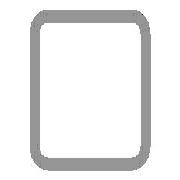
# Autodesk Inventor part: DD_KVD_003_02
Saved by Autodesk Inventor 2017.3 (Build 213256000, 256)
## iProperties
IsCustomPart: 1
Created: 2016-02-22
Part Number: DD_KVD_003_02
Material: Nerezová ocel
Description: Tenkostěnné profily ocelové svařované (čtvercový profil)
Document SubType Name: Plech
Standard: CSN 42 6935
Designer: Darena
Standards Organization: CSN
Language: cs-CZ
Size Designation: 35x35x3-875
Categories: <MemberInstance><Categories><Category DisplayName="Konstrukční profily" InternalName="089c4875-fa83-4c05-b084-43b9cc11f5ed" Mnemonic="GRDR"><CategoryParameter DisplayName="Hmotnost na délkovou jednotku" InternalName="0bb95a10-148f-4027-a459-38d7b056702a" Mnemonic="shpmass"/><CategoryParameter DisplayName="Plocha průřezu" InternalName="1ff91680-64b0-4202-b9a3-7fd3f94bba3b" Mnemonic="secarea"/><CategoryParameter DisplayName="Poloměr setrvačnosti (x)" InternalName="25778675-03e9-40c1-b6a8-4a9ed693320d" Mnemonic="gyrradx"/><CategoryParameter DisplayName="Modul pružnosti v kroucení" InternalName="26c1ec35-5026-4c63-ad0a-751cf684a536" Mnemonic="torrigmod"/><CategoryParameter DisplayName="Vzdálenost těžiště X-X" InternalName="26c9bdb8-9c79-4b4f-a92e-8e197583c9c4" Mnemonic="grcendistX"/><CategoryParameter DisplayName="Původní ID člena" InternalName="340afe4f-75d7-48d3-ab7d-943f3c3da468" Mnemonic="LegacyMemberID"/><CategoryParameter DisplayName="Délka základny" InternalName="42e34263-8f20-4d0e-ad48-bf1385b87c24" Mnemonic="shplen"/><CategoryParameter DisplayName="Moment setrvačnosti (y)" InternalName="4b9f58ea-bced-460e-81ea-3d29ca5a49e3" Mnemonic="inermomy"/><CategoryParameter DisplayName="Moment setrvačnosti (x)" InternalName="4cd780bc-73d7-43ac-917a-579e5cbd684d" Mnemonic="inermomx"/><CategoryParameter DisplayName="Uživatelský referenční bod" InternalName="4f1d1b73-316d-484b-a3df-9cbabb16eb77" Mnemonic="shpBasePoint"/><CategoryParameter DisplayName="Výška tvaru" InternalName="50274e7d-5ac0-4796-92cb-c59e54983c67" Mnemonic="shpheig"/><CategoryParameter DisplayName="Průřezový modul (y)" InternalName="59eaa5e9-d227-48dc-b6c1-6920f96e0f95" Mnemonic="secmody"/><CategoryParameter DisplayName="Označení průřezu" InternalName="5a64d034-428d-49c8-ba32-7619764de20f" Mnemonic="shpdes"/><CategoryParameter DisplayName="Průřezový modul (x)" InternalName="72cfad18-cf51-4ed4-aaa7-c6b224f8419f" Mnemonic="secmodx"/><CategoryParameter DisplayName="Průřezový modul pružnosti" InternalName="7c55a8dc-8844-49f9-a867-cc677b30ec9a" Mnemonic="torsecmod"/><CategoryParameter DisplayName="Šířka tvaru" InternalName="7c717d54-a18f-4666-b4d4-573cce22c62c" Mnemonic="shpwdth"/><CategoryParameter DisplayName="Druhá tloušťka tvaru" InternalName="9251a8e1-85fd-4e47-af99-afdb762317d9" Mnemonic="shpthick2"/><CategoryParameter DisplayName="Publikované popředí" InternalName="9c666724-f362-4ea7-ac62-f6a007de5c69" Mnemonic="shpFGAuto"/><CategoryParameter DisplayName="Vzdálenost těžiště Y-Y" InternalName="bcc4fb17-7af4-436a-8f8c-d0aa3b0248c5" Mnemonic="grcendistY"/><CategoryParameter DisplayName="Poloměr setrvačnosti (y)" InternalName="bfa18ebe-1636-4dbe-8d42-b263e0b73184" Mnemonic="gyrrady"/><CategoryParameter DisplayName="Tloušťka tvaru" InternalName="d109cf76-8eb4-42fc-9800-4409734adc67" Mnemonic="shpthick"/><CategoryParameter DisplayName="Koeficient deformace ve smyku" InternalName="de4c90c6-aaa8-468f-a335-6737b311b5d3" Mnemonic="shdispc"/><Category DisplayName="Trubky čtvercového/obdélníkového průřezu" InternalName="afc8e2d8-05d6-4609-8807-f98a9b7d2ed0" Mnemonic="SQRSHP"><CategoryParameter DisplayName="Plocha průřezu" InternalName="2f7f79dd-983c-4263-802a-5b6a1495fdc5" Mnemonic="secarea"/><CategoryParameter DisplayName="Průřezový modul (x)" InternalName="50d965a6-04bf-46b9-8ace-861858d348e6" Mnemonic="secmodx"/><CategoryParameter DisplayName="Průřezový modul (y)" InternalName="5106aeac-54a2-4159-a9af-8933dd39dba2" Mnemonic="secmody"/><CategoryParameter DisplayName="Tloušťka tvaru" InternalName="52712fc5-f4ee-4eda-b3f2-6fce82c26419" Mnemonic="shpthick"/><CategoryParameter DisplayName="Moment setrvačnosti (y)" InternalName="55ec8510-8276-4c45-8f10-594e0fee7eb3" Mnemonic="inermomy"/><CategoryParameter DisplayName="Poloměr setrvačnosti (x)" InternalName="56c89926-a299-4389-a862-ac94c9691272" Mnemonic="gyrradx"/><CategoryParameter DisplayName="Poloměr" InternalName="5d8d062c-e28e-41c1-98da-8e5fee36da1a" Mnemonic="shprad"/><CategoryParameter DisplayName="Moment setrvačnosti (x)" InternalName="8c4637b6-6b69-4878-9d5d-26a32185d655" Mnemonic="inermomx"/><CategoryParameter DisplayName="Šířka tvaru" InternalName="8c8a1782-5e80-4d77-858b-304b1c0ad1fd" Mnemonic="shpwdth"/><CategoryParameter DisplayName="Poloměr setrvačnosti (y)" InternalName="fa48a7f5-f030-40f9-a60b-de8a845b7104" Mnemonic="gyrrady"/></Category></Category><Category DisplayName="Typdat" InternalName="23b78d0f-2648-40c6-8793-ca6db495c9e8" Mnemonic="DATATYPE"><CategoryParameter DisplayName="Zobrazovanýnázev" InternalName="05415f3d-3907-474b-a020-eb9d644f4cf3" Mnemonic="DISPLAYNAME"/><CategoryParameter DisplayName="Norma" InternalName="0c0a119c-1e12-4c84-803f-101930972f5e" Mnemonic="STANDARD"/><CategoryParameter DisplayName="Popis" InternalName="13903e3d-64b1-4950-80da-f627842ea37f" Mnemonic="DESCRIPTION"/><CategoryParameter DisplayName="Označení" InternalName="2675968c-4ce5-49e0-a4f5-552d29089031" Mnemonic="DESIGNATION"/><CategoryParameter DisplayName="Výchozí řada" InternalName="2af9ec52-faaa-4026-b378-f9fa4afca842" Mnemonic="DEFAULTROW"/><CategoryParameter DisplayName="Název složky" InternalName="3f06958e-8713-4116-9be7-ed6184ecc97b" Mnemonic="FOLDERNAME"/><CategoryParameter DisplayName="GUID verze" InternalName="45a75005-10b1-4dfc-8d6d-dfe629f0b93c" Mnemonic="REVISIONGUID"/><CategoryParameter DisplayName="Názevsouboru" InternalName="8b46a4cc-9585-4fed-90c3-899f57e09a73" Mnemonic="FILENAME"/><CategoryParameter DisplayName="Normalizační institut" InternalName="8f5914e1-4693-403f-8ab5-d37768198c9d" Mnemonic="STDSORG"/><CategoryParameter DisplayName="Verze rodiny" InternalName="914462f6-6e19-4b14-ba84-155b9680b1d0" Mnemonic="FAMILYREVISION"/><CategoryParameter DisplayName="Revize normy" InternalName="91d5a463-65c2-4fde-b823-3b7fea5e8e17" Mnemonic="STANDARDREVISION"/><CategoryParameter DisplayName="Revize členu" InternalName="a65d44b9-392f-4f4f-857b-e4b3d54996fe" Mnemonic="MEMBERREVISION"/><CategoryParameter DisplayName="Formátoříznutí" InternalName="bc51e27b-3422-4e78-93ef-cec197ddf230" Mnemonic="CLIPFORMAT"/><CategoryParameter DisplayName="Výrobce" InternalName="cd6c7a72-a28a-4e50-99a9-2c7f4e13e5ad" Mnemonic="MANUFACTURER"/><CategoryParameter DisplayName="Internínázev" InternalName="cf1d0246-76d9-4b4a-8305-fa0409afb5c1" Mnemonic="INTERNALNAME"/><CategoryParameter DisplayName="Jemetrický" InternalName="e2385c5b-1ea4-4823-96a8-8de651266ec3" Mnemonic="ISMETRIC"/><Category DisplayName="Díl" InternalName="c0e0b642-3bcb-4cc8-9e80-f96d35c4afa4" Mnemonic="PART"><CategoryParameter DisplayName="Číslo dílu" InternalName="016b6077-bfbe-49bd-92c9-d8d59c39c941" Mnemonic="PARTNUMBER"/><CategoryParameter DisplayName="Skladové číslo" InternalName="4dba7c1c-e26c-444e-836c-b08b433409a8" Mnemonic="STOCKNUMBER"/><CategoryParameter DisplayName="Materiál pera" InternalName="5c9a8adb-dd2b-4535-b97f-0a94a95fe41f" Mnemonic="MATERIALKEY"/><CategoryParameter DisplayName="Materiál" InternalName="818a152a-d3c3-49ca-80ee-df7d91421b8e" Mnemonic="MATERIAL"/></Category></Category><Category DisplayName="Původní mapování DA" InternalName="924fff40-ddd0-4eff-ad42-30e3774ef79e" Mnemonic="LEGACYMAPDA"><CategoryParameter DisplayName="DACookie" InternalName="316934ee-8fe1-4c7a-9c36-f2d79e1add1a" Mnemonic="DACOOKIE"/></Category></Categories><FamilyTemplate Id="N426935"><FamilyTemplateParameters><FamilyTemplateParameter ObjectType="kUserParameterObject" ValueType="xs:integer" Id="1" ObjectReferenceKey="b"/><FamilyTemplateParameter ObjectType="kUserParameterObject" ValueType="xs:double" Id="2" ObjectReferenceKey="ParT"/><FamilyTemplateParameter ObjectType="kUserParameterObject" ValueType="xs:double" Id="3" ObjectReferenceKey="B_L"/><FamilyTemplateParameter ObjectType="kPropertyObject" ValueType="xs:string" Id="100" ObjectReferenceKey="{32853F0F-3444-11d1-9E93-0060B03C1CA6}" SubObjectId="52"/><FamilyTemplateParameter ObjectType="kPropertyObject" ValueType="xs:string" Id="105" ObjectReferenceKey="{32853F0F-3444-11d1-9E93-0060B03C1CA6}" SubObjectId="5"/><FamilyTemplateParameter ObjectType="kPartComponentDefinitionObject" ValueType="xs:string" Id="110" SubObjectId="Material"/><FamilyTemplateParameter ObjectType="kPropertyObject" ValueType="xs:string" Id="112" ObjectReferenceKey="{32853F0F-3444-11d1-9E93-0060B03C1CA6}" SubObjectId="55"/></FamilyTemplateParameters></FamilyTemplate><CategoryParameterMap><ParamToTemplateMap><ParamToTemplate CategoryParameter="//CategoryParameter[@InternalName='05415f3d-3907-474b-a020-eb9d644f4cf3']" ConstantValue="CSN 426935"/><ParamToTemplate CategoryParameter="//CategoryParameter[@InternalName='cf1d0246-76d9-4b4a-8305-fa0409afb5c1']" ConstantValue="C8A6E4F3-6C70-40B5-A76F-D38F9965835C"/><ParamToTemplate CategoryParameter="//CategoryParameter[@InternalName='3f06958e-8713-4116-9be7-ed6184ecc97b']" ConstantValue="CSN 426935"/><ParamToTemplate CategoryParameter="//CategoryParameter[@InternalName='914462f6-6e19-4b14-ba84-155b9680b1d0']" ConstantValue="10"/><ParamToTemplate CategoryParameter="//CategoryParameter[@InternalName='bc51e27b-3422-4e78-93ef-cec197ddf230']" ConstantValue="CF_INVENTOR.STDPARTS"/><ParamToTemplate CategoryParameter="//CategoryParameter[@InternalName='e2385c5b-1ea4-4823-96a8-8de651266ec3']" ConstantValue="true"/><ParamToTemplate CategoryParameter="//CategoryParameter[@InternalName='13903e3d-64b1-4950-80da-f627842ea37f']" ConstantValue="Steel thin-walled sections, welded (square  profile)"/><ParamToTemplate CategoryParameter="//CategoryParameter[@InternalName='8f5914e1-4693-403f-8ab5-d37768198c9d']" ConstantValue="CSN"/><ParamToTemplate CategoryParameter="//CategoryParameter[@InternalName='0c0a119c-1e12-4c84-803f-101930972f5e']" ConstantValue="CSN 42 6935"/><ParamToTemplate CategoryParameter="//CategoryParameter[@InternalName='cd6c7a72-a28a-4e50-99a9-2c7f4e13e5ad']" TemplateParameter="104"/><ParamToTemplate CategoryParameter="//CategoryParameter[@InternalName='91d5a463-65c2-4fde-b823-3b7fea5e8e17']" TemplateParameter="103"/><ParamToTemplate CategoryParameter="//CategoryParameter[@InternalName='45a75005-10b1-4dfc-8d6d-dfe629f0b93c']" ConstantValue="d63989c9-529b-4c73-9570-6fdae8f60a36"/><ParamToTemplate CategoryParameter="//CategoryParameter[@InternalName='2af9ec52-faaa-4026-b378-f9fa4afca842']" ConstantValue="10"/><ParamToTemplate CategoryParameter="//CategoryParameter[@InternalName='9c666724-f362-4ea7-ac62-f6a007de5c69']" ConstantValue="1"/><ParamToTemplate CategoryParameter="//CategoryParameter[@InternalName='8b46a4cc-9585-4fed-90c3-899f57e09a73']" ConstantValue="CSN 426935 - 35x35x3-875"/><ParamToTemplate CategoryParameter="//CategoryParameter[@InternalName='a65d44b9-392f-4f4f-857b-e4b3d54996fe']" ConstantValue="F905554A-FDA4-40BB-94B6-85A1861FF3FA"/><ParamToTemplate CategoryParameter="//CategoryParameter[@InternalName='8c4637b6-6b69-4878-9d5d-26a32185d655']" ConstantValue="57120"/><ParamToTemplate CategoryParameter="//CategoryParameter[@InternalName='50d965a6-04bf-46b9-8ace-861858d348e6']" ConstantValue="3264"/><ParamToTemplate CategoryParameter="//CategoryParameter[@InternalName='2f7f79dd-983c-4263-802a-5b6a1495fdc5']" ConstantValue="349,5"/><ParamToTemplate CategoryParameter="//CategoryParameter[@InternalName='7c55a8dc-8844-49f9-a867-cc677b30ec9a']" ConstantValue="4915,2"/><ParamToTemplate CategoryParameter="//CategoryParameter[@InternalName='26c1ec35-5026-4c63-ad0a-751cf684a536']" ConstantValue="78643,2"/><ParamToTemplate CategoryParameter="//CategoryParameter[@InternalName='de4c90c6-aaa8-468f-a335-6737b311b5d3']" ConstantValue="2,1"/><ParamToTemplate CategoryParameter="//CategoryParameter[@InternalName='316934ee-8fe1-4c7a-9c36-f2d79e1add1a']" ConstantValue="*CSN~N42 6935~35x35x3-25000*"/><ParamToTemplate CategoryParameter="//CategoryParameter[@InternalName='42e34263-8f20-4d0e-ad48-bf1385b87c24']" TemplateParameter="3"/><ParamToTemplate CategoryParameter="//CategoryParameter[@InternalName='2675968c-4ce5-49e0-a4f5-552d29089031']" TemplateParameter="100"/><ParamToTemplate CategoryParameter="//CategoryParameter[@InternalName='818a152a-d3c3-49ca-80ee-df7d91421b8e']" TemplateParameter="110"/><ParamToTemplate CategoryParameter="//CategoryParameter[@InternalName='016b6077-bfbe-49bd-92c9-d8d59c39c941']" TemplateParameter="105"/><ParamToTemplate CategoryParameter="//CategoryParameter[@InternalName='4dba7c1c-e26c-444e-836c-b08b433409a8']" TemplateParameter="112"/></ParamToTemplateMap></CategoryParameterMap></MemberInstance>
Stock Number: 35x35x3
Density: 8 g/cm^3
Appearance: Pololeštěná
Sheet Metal Rule: Výchozí
G_L: 875,000 mm
Author: Darena
Autodesk Inventor part; units mm, degrees
ref_plane "Počáteční rovina" through (0, 0, 0) normal (0, 0, 1) x (1, 0, 0)
ref_plane "Koncová rovina" through (0, 0, 875) normal (0, 0, 1) x (1, 0, 0)
sketch "Náčrt1" plane through (0, 0, 0) normal (0, 0, 1) x (1, 0, 0)
  line L0 (-11.5, 17.5) -> (11.5, 17.5)
  line L1 (17.5, 11.5) -> (17.5, -11.5)
  line L2 (11.5, -17.5) -> (-11.5, -17.5)
  line L3 (-17.5, -11.5) -> (-17.5, 11.5)
  arc A0 (-11.5, 17.5) -> (-17.5, 11.5) centre (-11.5, 11.5) ccw
  arc A1 (17.5, 11.5) -> (11.5, 17.5) centre (11.5, 11.5) ccw
  arc A2 (11.5, -17.5) -> (17.5, -11.5) centre (11.5, -11.5) ccw
  arc A3 (-17.5, -11.5) -> (-11.5, -17.5) centre (-11.5, -11.5) ccw
  line L4 (-26.2397, 0) -> (26.2397, 0) construction
  line L5 (0, -26.2397) -> (0, 26.2397) construction
  arc A4 (-11.5, 14.5) -> (-14.5, 11.5) centre (-11.5, 11.5) ccw
  line L6 (-11.5, 14.5) -> (11.5, 14.5)
  arc A5 (14.5, 11.5) -> (11.5, 14.5) centre (11.5, 11.5) ccw
  line L7 (14.5, 11.5) -> (14.5, -11.5)
  arc A6 (11.5, -14.5) -> (14.5, -11.5) centre (11.5, -11.5) ccw
  line L8 (11.5, -14.5) -> (-11.5, -14.5)
  arc A7 (-14.5, -11.5) -> (-11.5, -14.5) centre (-11.5, -11.5) ccw
  line L9 (-14.5, -11.5) -> (-14.5, 11.5)
  point P0 (-17.5, 17.5)
  point P1 (17.5, -17.5)
  point P2 (17.5, 17.5)
  dimension "b" = 35
  dimension "msp_r" = 6
  dimension "d8" = 17.5
  dimension "d9" = 17.5
  dimension "d10" = 3
  constraints: 16 end point, 16 point on circle, 8 centre point, 8 tangent, 6 point on line, 4 parallel, 3 equal radius, 3 perpendicular, 1 horizontal, 7 other
  measures "b" distance of point (-17.5, 17.5) point (17.5, 17.5)
  measures "msp_r" radius of A0
  measures "d8" distance between parallel lines of L3 L5
  measures "d9" distance between parallel lines of L2 L4
  measures "d10" distance between parallel lines of L2 L8
extrude "Těleso" add sketch "Náčrt1" along normal blind 870
sketch "Sketch2" plane through (0, 0, 0) normal (0, 0, 1) x (1, 0, 0)
  line L0 (0, 0) -> (10, 0)
ref_plane "Work Plane3" through (0, 0, 0) normal (0, -1, 0) x (1, 0, 0)
sketch "Sketch3" plane through (0, 0, 0) normal (0, -1, 0) x (1, 0, 0)
  line L0 (-2, 0) -> (12, 0)
  line L1 (-2, 875) -> (12, 875)
  dimension "d14" = 875
  measures "d14" distance between parallel lines of L0 L1
sketch "Náčrt4" plane through (11.5, 17.5, 875) normal (0, 1, 0) x (1, 0, 0)
  line L0 (-29, 875) -> (-29, 5) construction
  line L1 (6, 875) -> (6, 5) construction
  line L2 (-29, 875) -> (6, 875)
  line L3 (6, 875) -> (6, 840)
  line L4 (-29, 875) -> (-29, 5) construction
  line L5 (6, 840) -> (-29, 875)
  line L6 (6, 875) -> (6, 5) construction
  line L7 (-23, 5) -> (-29, 5) projected
  line L8 (-29, 5) -> (6, 40)
  line L9 (6, 40) -> (6, 5)
  line L10 (6, 5) -> (-29, 5)
  point P0 (-11.5, 875)
  dimension "d15" = 45
  dimension "d19" = 45
  constraints: 12 end point, 2 point on line, 1 collinear, 1 horizontal, 1 perpendicular
  measures "d15" angle of L5 L2
  measures "d19" angle of L10 L8
extrude "Vysunutí2" cut sketch "Náčrt4" against normal through all
ref_plane "Pracovní rovina4" through (417.5, -11.5, 435) normal (0, 0, 1) x (0, -1, 0)
equation "\"msp_r\" = 2 * ParT"
equation "\"d8\" = d9"
equation "\"d9\" = 0.5 * b"
equation "\"d10\" = ParT"
equation "\"G_OFFSET_START\" = 0"
equation "\"G_OFFSET_END\" = 0"
equation "\"d12\" = G_OFFSET_END + B_L"
equation "\"G_L\" = d14"
equation "\"B_L\" = 875"
equation "\"PoloměrOhybu\" = Tloušťka"
equation "\"ŠířkaVýštipu\" = Tloušťka"
equation "\"HloubkaVýštipu\" = 0.5 * Tloušťka"
equation "\"VelikostRohovéhoVýštipu\" = 4 * Tloušťka"
equation "\"MinimálníZbytek\" = 2 * Tloušťka"
equation "\"PřechodovýPoloměr\" = PoloměrOhybu"
equation "\"VelikostJacobihoPoloměru\" = Tloušťka"
equation "\"VelikostMezery\" = Tloušťka"
equation "\"ParT\" = 3"
equation "\"Tloušťka\" = 0.5"
body "Solid1"
